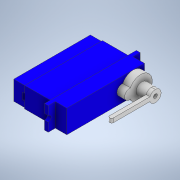
# Autodesk Inventor part: Servomotor1
Saved by Autodesk Inventor 2022 (Build 260153000, 153)
## iProperties
Created: 2021-07-03
Part Number: Servomotor1
Material: Generic
Document SubType Name: Modeling
Designer: Bhagiratha
Density: 1 g/cm^3
Appearance: Default
Author: Bhagiratha
Autodesk Inventor part; units mm, degrees
ref_plane "YZ Plane" through (0, 0, 0) normal (1, 0, 0) x (0, 1, 0)
ref_plane "XZ Plane" through (0, 0, 0) normal (0, 1, 0) x (-1, 0, 0)
ref_plane "XY Plane" through (0, 0, 0) normal (0, 0, 1) x (1, 0, 0)
sketch "Sketch1" plane through (0, 0, 0) normal (1, 0, 0) x (0, 1, 0)
  line L0 (-25, 100) -> (25, 100)
  line L1 (25, 100) -> (25, -100)
  line L2 (25, -100) -> (-25, -100)
  line L3 (-25, -100) -> (-25, 100)
  line L4 (-25, 100) -> (25, -100) construction
  line L5 (25, 100) -> (-25, -100) construction
  point P0 (0, 0)
  dimension "d0" = 50
  dimension "d1" = 200
  constraints: 12 end point, 2 midpoint, 2 parallel, 1 horizontal, 1 perpendicular
  measures "d0" distance of L1.end L2.end
  measures "d1" distance of L0.end L1.end
extrude "Extrusion1" add sketch "Sketch1" along normal blind 30
sketch "Sketch2" plane through (30, 0, 0) normal (1, 0, 0) x (0, 0, -1)
  line L0 (101.5, -26.5) -> (-101.5, -26.5)
  line L1 (-101.5, -26.5) -> (-101.5, 26.5)
  line L2 (-101.5, 26.5) -> (101.5, 26.5)
  line L3 (101.5, 26.5) -> (101.5, -26.5)
  line L4 (101.5, -26.5) -> (-101.5, 26.5) construction
  line L5 (-101.5, -26.5) -> (101.5, 26.5) construction
  point P0 (0, 0)
  dimension "d4" = 203
  dimension "d5" = 53
  constraints: 12 end point, 2 midpoint, 2 parallel, 1 horizontal, 1 perpendicular
  measures "d4" distance of L1.end L2.end
  measures "d5" distance of L0.end L1.end
extrude "Extrusion2" add sketch "Sketch2" along normal blind 70
sketch "Sketch3" plane through (100, 0, 0) normal (1, 0, 0) x (0, 0, -1)
  line L0 (120, 30) -> (-120, 30)
  line L1 (-120, 30) -> (-120, -30)
  line L2 (-120, -30) -> (120, -30)
  line L3 (120, -30) -> (120, 30)
  line L4 (120, 30) -> (-120, -30) construction
  line L5 (-120, 30) -> (120, -30) construction
  point P0 (0, 0)
  dimension "d8" = 240
  dimension "d9" = 60
  constraints: 12 end point, 2 midpoint, 2 parallel, 1 horizontal, 1 perpendicular
  measures "d8" distance of L2.end L1.end
  measures "d9" distance of L1.end L0.end
extrude "Extrusion3" add sketch "Sketch3" along normal blind 10
sketch "Sketch4" plane through (110, 0, 0) normal (1, 0, 0) x (0, 0, -1)
  line L0 (101.5, -30) -> (-101.5, -30)
  line L1 (-101.5, -30) -> (-101.5, 30)
  line L2 (-101.5, 30) -> (101.5, 30)
  line L3 (101.5, 30) -> (101.5, -30)
  line L4 (101.5, -30) -> (-101.5, 30) construction
  line L5 (-101.5, -30) -> (101.5, 30) construction
  point P0 (0, 0)
  dimension "d12" = 203
  dimension "d13" = 60
  constraints: 12 end point, 2 midpoint, 2 parallel, 1 horizontal, 1 perpendicular
  measures "d12" distance of L1.end L2.end
  measures "d13" distance of L0.end L1.end
extrude "Extrusion4" add sketch "Sketch4" along normal blind 30
sketch "Sketch6" plane through (140, 0, 0) normal (1, 0, 0) x (0, 0, -1)
  arc A0 (44.5, -13.0767) -> (44.5, 13.0767) centre (71.5, 0) ccw
  line L0 (101.5, -30) -> (101.5, 30) projected
  arc A1 (44.5, 13.0767) -> (44.5, -13.0767) centre (42.5487, 0) ccw
  point P0 (0, 0)
  point P1 (44.5, 13.0767)
  dimension "d16" = 60
  dimension "d17" = 30
  constraints: 4 point on circle, 2 centre point
  measures "d16" diameter of A0
  measures "d17" distance from line of L0 A0.centre
extrude "Extrusion5" add sketch "Sketch6" along normal blind 20
sketch "Sketch8" plane through (160, 0, 0) normal (1, 0, 0) x (0, 0, -1)
  circle A0 centre (71.456, 0) radius 7.5
  point P0 (0, 0)
  dimension "d22" = 15
  constraints: 1 centre point
  measures "d22" diameter of A0
extrude "Extrusion6" add sketch "Sketch8" along normal blind 3
sketch "Sketch9" plane through (163, 0, -71.456) normal (1, 0, 0) x (0, 0, -1)
  circle A0 centre (0, 0) radius 15
  point P0 (-71.456, 0)
  dimension "d25" = 30
  constraints: 1 centre point
  measures "d25" diameter of A0
extrude "Extrusion7" add sketch "Sketch9" along normal blind 25
sketch "Sketch10" plane through (188, 0, -71.456) normal (1, 0, 0) x (0, 0, -1)
  circle A0 centre (0, 0) radius 7.5 projected
  circle A1 centre (0, 0) radius 5
  point P0 (-71.456, 0)
  dimension "d28" = 10
  constraints: 1 centre point, 1 coincident
  measures "d28" diameter of A1
extrude "Extrusion8" cut sketch "Sketch10" against normal blind 25 contours A0 | A1
sketch "Sketch11" plane through (188, 0, -71.456) normal (1, 0, 0) x (0, 0, -1)
  arc A0 (-13.9898, -5.3852) -> (-13.9898, 5.3852) centre (0.0102, 0) ccw
  circle A1 centre (0, 0) radius 15 projected
  line L0 (-13.9898, 5.4117) -> (-13.9898, 5.3852)
  line L1 (-13.9898, -5.3852) -> (-13.9898, -5.4117)
  line L2 (-13.9898, 5.3852) -> (-113.9898, 5.3852)
  line L3 (-113.9898, 5.3852) -> (-113.9898, -5.3852)
  line L4 (-113.9898, -5.3852) -> (-13.9898, -5.3852)
  point P0 (-71.456, 0)
  point P1 (0.0051, -15)
  point P2 (0.0051, 15)
  dimension "d31" = 30
  dimension "d38" = 100
  dimension "d39" = 10.7703
  constraints: 10 end point, 4 point on circle, 2 perpendicular, 2 vertical, 1 centre point, 1 horizontal
  measures "d31" diameter of A0
  measures "d38" distance of L3.end L1.start
  measures "d39" distance of L2.end L3.end
extrude "Extrusion9" add sketch "Sketch11" along normal blind 10 separate body contours L4 A1 L2 A0 | A0 A1 L1 | A1 A0 | L4 L3 L2 A1 | A0 L0 A1
sketch "Sketch12" plane through (198, 0, -71.456) normal (1, 0, 0) x (0, 0, -1)
  circle A0 centre (0, 0) radius 5
  point P0 (-71.456, 0)
  dimension "d37" = 10
  constraints: 1 centre point
  measures "d37" diameter of A0
extrude "Extrusion10" cut sketch "Sketch12" against normal blind 10 bodies 2
fillet "Fillet1" radius 5 2 edges at (198, 0, 42.5338) (188, 0, 42.5338)
sketch "Sketch13" plane through (110, 0, 0) normal (1, 0, 0) x (0, 0, -1)
  line L0 (120, -30) -> (120, 30) projected
  circle A0 centre (120, 0) radius 7.5
  line L1 (-120, 30) -> (-120, -30) projected
  circle A1 centre (-120, 0) radius 7.5
  point P0 (0, 0)
  dimension "d41" = 15
  dimension "d42" = 15
  constraints: 2 centre point, 2 midpoint
  measures "d41" diameter of A0
  measures "d42" diameter of A1
extrude "Extrusion11" cut sketch "Sketch13" against normal through all bodies 1
sketch "Sketch14" plane through (0, -25, -100) normal (0, 0, -1) x (-1, 0, 0)
  line L0 (-30, 50) -> (-30, 0) projected
  line L1 (-30, 14.331) -> (-23, 14.331)
  line L2 (-23, 14.331) -> (-23, 32.331)
  line L3 (-23, 32.331) -> (-30, 32.331)
  line L4 (-30, 32.331) -> (-30, 14.331)
  point P0 (0, 25)
  dimension "d45" = 7
  dimension "d46" = 18
  constraints: 8 end point, 2 parallel, 1 horizontal, 1 perpendicular, 1 point on line
  measures "d45" distance of L3.end L2.end
  measures "d46" distance of L2.end L1.end
extrude "Extrusion12" cut sketch "Sketch14" against normal through all bodies 1
body "Solid1"
body "Solid2"
